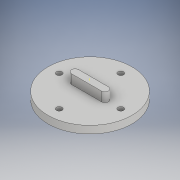
# Autodesk Inventor part: motormount_v3_richard
Saved by Autodesk Inventor 2018 (Build 220112000, 112)
## iProperties
Created: 2017-05-01
Part Number: motormount_v3_richard
Material: Generic
Document SubType Name: Modeling
Designer: mundhend06
Density: 1 g/cm^3
Appearance: Default
Author: mundhend06
Autodesk Inventor part; units mm, degrees
ref_plane "YZ Plane" through (0, 0, 0) normal (1, 0, 0) x (0, 1, 0)
ref_plane "XZ Plane" through (0, 0, 0) normal (0, 1, 0) x (-1, 0, 0)
ref_plane "XY Plane" through (0, 0, 0) normal (0, 0, 1) x (1, 0, 0)
sketch "Sketch1" plane through (0, 0, 0) normal (0, 1, 0) x (-1, 0, 0)
  circle A0 centre (0, 0) radius 22.5
  dimension "d0" = 45
  constraints: 1 centre point, 1 coincident
  measures "d0" diameter of A0
extrude "Extrusion1" add sketch "Sketch1" along normal blind 4
sketch "Sketch2" plane through (0, 4, 0) normal (0, 1, 0) x (1, 0, 0)
  line L0 (0, 0) -> (0, 8) construction
  line L1 (0, 0) -> (0, -8) construction
  circle A0 centre (0, 8) radius 1.9
  circle A1 centre (0, 0) radius 1.9
  circle A2 centre (0, -8) radius 1.9
  line L2 (1.9, 0) -> (1.9, -8)
  line L3 (1.9, 0) -> (1.9, 8)
  line L4 (-1.9, -8) -> (-1.9, 0)
  line L5 (-1.9, 0) -> (-1.9, 8)
  dimension "d3" = 8
  dimension "d4" = 8
  dimension "d5" = 3.8
  dimension "d6" = 3.8
  dimension "d7" = 3.8
  constraints: 12 end point, 6 point on circle, 3 centre point, 3 coincident, 3 vertical, 2 point on line, 2 tangent
  measures "d3" distance of L0.start L0.end
  measures "d4" distance of L0.start L1.end
  measures "d5" diameter of A0
  measures "d6" diameter of A1
  measures "d7" diameter of A2
extrude "Extrusion2" add sketch "Sketch2" along normal blind 5
sketch "Sketch7" plane through (0, 0, 0) normal (0, -1, 0) x (1, 0, 0)
  circle A0 centre (0, 0) radius 16.5 construction
  circle A1 centre (0, 16.5) radius 1.5
  circle A2 centre (16.5, 0) radius 1.5
  circle A3 centre (-16.5, 0) radius 1.5
  circle A4 centre (0, -16.5) radius 1.5
  dimension "d42" = 33
  dimension "d43" = 3
  dimension "d44" = 3
  dimension "d45" = 3
  dimension "d46" = 3
  constraints: 5 centre point, 4 point on circle, 1 coincident
  measures "d42" diameter of A0
  measures "d43" diameter of A1
  measures "d44" diameter of A2
  measures "d45" diameter of A3
  measures "d46" diameter of A4
extrude "Extrusion6" cut sketch "Sketch7" against normal blind 5
body "Solid1"
